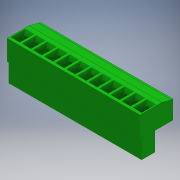
# Autodesk Inventor part: OST_OSTJ125153
Saved by Autodesk Inventor 2018 (Build 220112000, 112)
## iProperties
Created: 2018-11-13
Part Number: OST_OSTJ125153
Material: Polypropylene
Document SubType Name: Modeling
Designer: Rich
Density: 0.899 g/cm^3
Appearance: Dark Green
MFG: ON SHORE TECH
MPN: OSTTJ125153
PRICE: 5.71
VENDOR: DIGIKEY
VPN: ED2905-ND
Author: Rich
Autodesk Inventor part; units mm, degrees
ref_plane "YZ Plane" through (0, 0, 0) normal (1, 0, 0) x (0, 1, 0)
sketch "Sketch1" plane through (0, 0, 0) normal (1, 0, 0) x (0, 1, 0)
  line L0 (-3.75, 0.4) -> (-3.75, 9.6)
  line L1 (-3.75, 9.6) -> (6.25, 9.6)
  line L2 (11.35, 8.4344) -> (11.35, 0)
  line L3 (11.35, 0) -> (3, 0)
  line L4 (3, 0) -> (3, -8.6)
  line L5 (3, -8.6) -> (-3, -8.6)
  line L6 (-3, -8.6) -> (-3, 0.4)
  line L7 (-3, 0.4) -> (-3.75, 0.4)
  line L8 (17.5, 0) -> (-17.5, 0) construction
  line L9 (0, -17.5) -> (0, 17.5) construction
  line L10 (0, -8.6) -> (0, 9.6) construction
  line L11 (6.25, 9.6) -> (10.6, 8.4344)
  line L12 (10.6, 8.4344) -> (11.35, 8.4344)
  point P0 (0, 0)
  point P1 (0, 0)
  dimension "d3" = 8.6
  dimension "d4" = 18.2
  dimension "d5" = 15.1
  dimension "d6" = 165
  dimension "d7" = 0.75
  dimension "d8" = 6
  dimension "d9" = 9.2
  dimension "d10" = 0.75
  dimension "d11" = 35
  dimension "d12" = 10
  constraints: 26 end point, 10 perpendicular, 3 midpoint, 3 point on line, 2 vertical, 1 coincident, 1 horizontal
  measures "d3" distance of L3.end L4.end
  measures "d4" vertical distance of L5.end L0.end
  measures "d5" horizontal distance of L0.end L2.start
  measures "d6" angle of L1 L11
  measures "d7" distance of L11.end L2.start
  measures "d8" distance of L4.end L5.end
  measures "d9" distance of L0.start L0.end
  measures "d10" distance between parallel lines of L0 L6
  measures "d11" distance of L8.start L8.end
  measures "d12" distance of L0.end L1.end
extrude "Extrusion1" add sketch "Sketch1" along normal blind 60.96
sketch "Sketch2" plane through (0, -3.75, 9.6) normal (0, 0, 1) x (1, 0, 0)
  line L0 (0, 0) -> (0, 10) construction
  line L1 (0, 0) -> (60.96, 0) construction
  line L2 (60.96, 10) -> (60.96, 0) construction
  line L3 (0, 10) -> (60.96, 10) construction
  line L4 (0, 3.8) -> (60.96, 3.8) construction
  line L5 (1.04, 5.8) -> (4.04, 5.8)
  line L6 (4.04, 5.8) -> (4.04, 1.8)
  line L7 (4.04, 1.8) -> (1.04, 1.8)
  line L8 (1.04, 1.8) -> (1.04, 5.8)
  line L9 (1.04, 5.8) -> (4.04, 1.8) construction
  line L10 (4.04, 5.8) -> (1.04, 1.8) construction
  point P0 (0, 3.75)
  point P1 (2.54, 3.8)
  dimension "d15" = 2.54
  dimension "d16" = 3
  dimension "d17" = 4
  dimension "d25" = 3.8
  constraints: 14 end point, 3 point on line, 2 midpoint, 2 parallel, 2 perpendicular, 1 horizontal
  measures "d15" distance of L4.start point (2.54, 3.8)
  measures "d16" distance of L5.start L5.end
  measures "d17" distance of L5.end L6.end
  measures "d25" distance between parallel lines of L1 L4
extrude "Extrusion2" cut sketch "Sketch2" against normal blind 10
sketch "Sketch3" plane through (0, -3, -8.6) normal (0, 0, -1) x (-1, 0, 0)
  line L0 (-4.04, 5.05) -> (-4.04, 1.05) construction
  line L1 (-1.04, 5.05) -> (-4.04, 5.05) construction
  line L2 (-4.04, 1.05) -> (-1.04, 1.05) construction
  line L3 (-1.04, 1.05) -> (-1.04, 5.05) construction
  line L4 (-4.04, 5.05) -> (-1.04, 1.05) construction
  line L5 (-1.04, 5.05) -> (-4.04, 1.05) construction
  circle A0 centre (-2.54, 3.05) radius 0.9
  point P0 (0, 3)
  dimension "d28" = 1.8
  constraints: 4 end point, 1 centre point, 1 midpoint
  measures "d28" diameter of A0
extrude "Extrusion3" cut sketch "Sketch3" against normal up to next
chamfer "Chamfer1" distance 2 distance2 4 1 edges at (2.54, 2.05, 9.6) measured on face at (41.9867, 1.5167, 9.6)
chamfer "Chamfer2" distance 0.5 distance2 4 1 edges at (1.04, 0.05, 9.6) measured on face at (41.9867, 1.5167, 9.6)
chamfer "Chamfer3" distance 0.5 distance2 4 1 edges at (2.54, -1.95, 9.6) measured on face at (41.9867, 1.5167, 9.6)
chamfer "Chamfer4" distance 0.5 distance2 4 1 edges at (4.04, 0.05, 9.6) measured on face at (41.9867, 1.5167, 9.6)
sketch "Sketch4" plane through (0, 11.35, 8.4344) normal (0, 1, 0) x (1, 0, 0)
  line L0 (0, 0) -> (0, 8.4344) construction
  line L1 (0, 0) -> (60.96, 0) construction
  line L2 (60.96, 8.4344) -> (60.96, 0) construction
  line L3 (0, 8.4344) -> (60.96, 8.4344) construction
  line L4 (0, 4.3344) -> (60.96, 4.3344) construction
  circle A0 centre (2.54, 4.3344) radius 1.75
  line L5 (0, -1.1656) -> (60.96, -1.1656) construction
  line L6 (1.29, 2.0094) -> (3.79, 2.0094)
  line L7 (3.79, 2.0094) -> (3.79, 0.7394)
  line L8 (3.79, 0.7394) -> (1.29, 0.7394)
  line L9 (1.29, 0.7394) -> (1.29, 2.0094)
  line L10 (1.29, 2.0094) -> (3.79, 0.7394) construction
  line L11 (3.79, 2.0094) -> (1.29, 0.7394) construction
  line L12 (2.54, 4.3344) -> (2.54, 1.3744) construction
  point P0 (0, 8.4344)
  dimension "d46" = 5.5
  dimension "d47" = 2.54
  dimension "d48" = 2.5
  dimension "d49" = 1.27
  dimension "d50" = 2.54
  dimension "d51" = 3.5
  constraints: 16 end point, 3 point on line, 2 horizontal, 2 midpoint, 2 parallel, 2 perpendicular, 1 centre point
  measures "d46" distance between parallel lines of L4 L5
  measures "d47" distance from line of L0 L12.start
  measures "d48" distance of L7.end L8.end
  measures "d49" distance of L6.end L7.end
  measures "d50" distance from line of L5 L12.end
  measures "d51" diameter of A0
extrude "Extrusion4" cut sketch "Sketch4" against normal blind 10
ref_plane "Work Plane1" through (50.8, 0, 0) normal (1, 0, 0) x (0, 0, -1)
sketch "Sketch6" plane through (50.8, 0, 0) normal (1, 0, 0) x (0, 0, -1)
  line L0 (-9.6, -3.75) -> (-0.4, -3.75) construction
  line L1 (-0.4, -3.75) -> (-0.4, -3) construction
  line L2 (-0.4, -3) -> (8.6, -3) construction
  line L3 (8.6, -3) -> (8.6, 3) construction
  line L4 (8.6, 3) -> (0, 3) construction
  line L5 (0, 3) -> (0, 11.35) construction
  line L6 (0, 11.35) -> (-8.4344, 11.35) construction
  line L7 (-8.4344, 11.35) -> (-8.4344, 10.6) construction
  line L8 (-8.4344, 10.6) -> (-9.6, 6.25) construction
  line L9 (-9.6, 6.25) -> (-9.6, -3.75) construction
  line L10 (0, 11.35) -> (0, 3) projected
  line L11 (0, 9.8084) -> (5.1352, 7.8094)
  line L12 (5.1352, 7.8094) -> (5.8305, 6.5927)
  line L13 (5.8305, 6.5927) -> (4.4979, 5.5787)
  line L14 (4.4979, 5.5787) -> (3.5419, 6.25)
  line L15 (3.5419, 6.25) -> (0, 7.175)
  line L16 (0, 9.8084) -> (0, 7.175)
  point P0 (0, 0)
  constraints: 12 end point, 1 collinear, 1 midpoint, 1 point on line
extrude "Extrusion5" add sketch "Sketch6" along normal blind 2.54
ref_plane "Work Plane2" through (30.48, 0, 0) normal (1, 0, 0) x (0, 0, -1)
mirror "Mirror1" about plane through (30.48, 0, 0) normal (1, 0, 0) of "Extrusion5"
pattern_linear "Rectangular Pattern1" count 12 spacing 5.08 along (1, 0, 0) of "Extrusion2", "Chamfer2", "Chamfer3", "Chamfer1", "Chamfer4", "Extrusion3", "Extrusion4"
body "Solid1"
